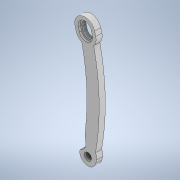
# Autodesk Inventor part: Part2
Saved by Autodesk Inventor 2020.3 (Build 243373000, 373)
## iProperties
Created: 2019-08-12
Part Number: Part2
Material: Generic
Document SubType Name: Modeling
Designer: Horváth Patrik
Density: 1 g/cm^3
Appearance: Default
Author: Horváth Patrik
Autodesk Inventor part; units mm, degrees
ref_plane "YZ Plane" through (0, 0, 0) normal (1, 0, 0) x (0, 1, 0)
ref_plane "XZ Plane" through (0, 0, 0) normal (0, 1, 0) x (-1, 0, 0)
ref_plane "XY Plane" through (0, 0, 0) normal (0, 0, 1) x (1, 0, 0)
ref_plane "Work Plane1" through (-0.0405, 69.8618, 0) normal (0, 0, 1) x (0.6413599, 0.7672402, 0)
ref_plane "Work Plane3" through (5.5931, 11.378, 1) normal (0, 0, 1) x (1, 0, 0)
sketch "Sketch2" plane through (5.5931, 11.378, 1) normal (0, 0, 1) x (1, 0, 0)
  arc A0 (-2.9323, 0.6339) -> (-4.1247, 52.0744) centre (-110.4489, 23.8756) ccw projected
  arc A1 (2.9323, -0.6339) -> (1.6748, 53.6125) centre (-110.4489, 23.8756) ccw projected
  arc A2 (1.6748, 53.6125) -> (-4.1247, 52.0744) centre (-1.225, 52.8435) ccw projected
  circle A3 centre (0, 0) radius 3 projected
  circle A4 centre (0, 0) radius 1.25 projected
  circle A5 centre (-1.225, 52.8435) radius 3 projected
  circle A6 centre (-1.225, 52.8435) radius 1.4795 projected
  point P0 (-5.5931, -11.378)
  point P1 (-2.9323, 0.6339)
  point P2 (2.9323, -0.6339)
extrude "Extrusion2" add sketch "Sketch2" along normal blind 3
ref_plane "Work Plane6" through (4.3681, 64.2214, 5) normal (0, 0, 1) x (1, 0, 0)
sketch "Sketch4" plane through (4.3681, 64.2214, 4) normal (0, 0, 1) x (1, 0, 0)
  arc A0 (4.1572, -53.4773) -> (2.8997, 0.7691) centre (-109.2239, -28.9678) ccw construction
  arc A1 (-1.7073, -52.2096) -> (-2.8997, -0.7691) centre (-109.2239, -28.9678) ccw construction
  circle A2 centre (0, 0) radius 3 construction
  circle A3 centre (0, 0) radius 3 construction
  circle A4 centre (0, 0) radius 1.4795 construction
  arc A5 (0.2521, -0.9677) -> (-0.2606, 0.9654) centre (-109.2239, -28.9678) ccw construction
  arc A6 (5.0961, 0.2712) -> (4.5608, 2.2899) centre (-109.2239, -28.9678) ccw
  arc A7 (-4.592, -2.2067) -> (-5.082, -0.359) centre (-109.2239, -28.9678) ccw
  arc A8 (-4.592, -2.2067) -> (5.0961, 0.2712) centre (0.2521, -0.9677) ccw
  arc A9 (4.5608, 2.2899) -> (-5.082, -0.359) centre (-0.2606, 0.9654) ccw
  arc A10 (-1.7073, -52.2096) -> (4.1572, -53.4773) centre (1.225, -52.8435) ccw projected
  arc A11 (2.8997, 0.7691) -> (-2.8997, -0.7691) centre (0, 0) ccw projected
  arc A12 (-1.7073, -52.2096) -> (-2.8997, -0.7691) centre (-109.2239, -28.9678) ccw projected
  point P0 (-4.3681, -64.2214)
  dimension "d16" = 10
  dimension "d26" = 1
  dimension "d27" = 1
  constraints: 11 point on circle, 5 centre point, 4 tangent, 2 coincident, 2 concentric
  measures "d16" radial gap between concentric circles of A7 A6
  measures "d26" distance of point (0, 0) A5.end
  measures "d27" distance of A5.start point (0, 0)
extrude "Extrusion4" add sketch "Sketch4" against normal blind 3
ref_plane "Work Plane7" through (5.5931, 11.378, 5) normal (0, 0, 1) x (1, 0, 0)
sketch "Sketch5" plane through (5.5931, 11.378, 5) normal (0, 0, 1) x (1, 0, 0)
  arc A0 (-0.9646, 51.8435) -> (-1.4951, 53.8435) centre (-110.4489, 23.8756) ccw construction
  arc A1 (0.7309, 52.2766) -> (0.1923, 54.3076) centre (-110.4489, 23.8756) ccw
  arc A2 (-2.6602, 51.4103) -> (-3.1824, 53.3794) centre (-110.4489, 23.8756) ccw
  arc A3 (-2.6602, 51.4103) -> (0.7309, 52.2766) centre (-0.9646, 51.8435) ccw
  arc A4 (0.1923, 54.3076) -> (-3.1824, 53.3794) centre (-1.4951, 53.8435) ccw
  arc A5 (2.6687, 52.7716) -> (2.1206, 54.838) centre (-110.4489, 23.8756) ccw projected
  arc A6 (2.1206, 54.838) -> (-5.1108, 52.849) centre (-1.4951, 53.8435) ccw projected
  arc A7 (-4.598, 50.9153) -> (-5.1108, 52.849) centre (-110.4489, 23.8756) ccw projected
  arc A8 (-4.598, 50.9153) -> (2.6687, 52.7716) centre (-0.9646, 51.8435) ccw projected
  arc A9 (3.3358, 55.1334) -> (-6.307, 52.4844) centre (-1.4856, 53.8089) ccw projected
  arc A10 (3.8712, 53.1147) -> (3.3358, 55.1334) centre (-110.4489, 23.8756) ccw projected
  arc A11 (2.869, 48.6758) -> (3.8712, 53.1147) centre (-0.9729, 51.8758) ccw projected
  arc A12 (-5.817, 50.6368) -> (-2.9702, 47.292) centre (-0.9729, 51.8758) ccw projected
  arc A13 (-5.817, 50.6368) -> (-6.307, 52.4844) centre (-110.4489, 23.8756) ccw projected
  point P0 (-5.5931, -11.378)
  dimension "d12" = 3.5
  constraints: 10 point on circle, 5 centre point, 4 tangent, 2 coincident, 2 concentric
  measures "d12" radial gap between concentric circles of A1 A2
extrude "Extrusion5" cut sketch "Sketch5" against normal blind 5 contours A3 A2 A4 A1
sketch "Sketch7" plane through (5.5931, 11.378, 4) normal (0, 0, 1) x (1, 0, 0)
  circle A0 centre (0, 0) radius 1.25 projected
  circle A1 centre (0, 0) radius 1.8
  arc A2 (-3.9097, 0.8452) -> (3.9097, -0.8452) centre (0, 0) ccw
  arc A3 (4.2266, 0.621) -> (-3.5928, 2.3113) centre (0.3169, 1.4661) ccw
  arc A4 (-2.9323, 0.6339) -> (-2.9702, 47.292) centre (-110.4489, 23.8756) ccw projected
  arc A5 (2.9323, -0.6339) -> (2.869, 48.6758) centre (-110.4489, 23.8756) ccw projected
  line L0 (0.3169, 1.4661) -> (0, 0) construction
  line L1 (-3.5928, 2.3113) -> (-3.9097, 0.8452)
  line L2 (4.2266, 0.621) -> (3.9097, -0.8452)
  line L3 (-2.9323, 0.6339) -> (2.9323, -0.6339) construction
  point P0 (-5.5931, -11.378)
  dimension "d19" = 3.6
  dimension "d20" = 8
  dimension "d21" = 1.5
  constraints: 8 end point, 4 point on circle, 4 tangent, 3 centre point, 2 coincident, 1 equal radius, 1 perpendicular
  measures "d19" diameter of A1
  measures "d20" diameter of A2
  measures "d21" distance of L0.start L0.end
extrude "Extrusion6" cut sketch "Sketch7" against normal up to surface (3 mm away) contours A1
extrude "Extrusion7" add sketch "Sketch7" against normal up to surface (3 mm away) contours L1 A3 L2 A2
sketch "Sketch8" plane through (5.5931, 11.378, 4) normal (0, 0, 1) x (1, 0, 0)
  arc A0 (-2.6602, 51.4103) -> (-3.1824, 53.3794) centre (-110.4489, 23.8756) ccw projected
  arc A1 (0.1923, 54.3076) -> (-3.1824, 53.3794) centre (-1.4951, 53.8435) ccw projected
  arc A2 (0.7309, 52.2766) -> (0.1923, 54.3076) centre (-110.4489, 23.8756) ccw projected
  arc A3 (-2.6602, 51.4103) -> (0.7309, 52.2766) centre (-0.9646, 51.8435) ccw projected
  arc A4 (-3.3868, 51.2247) -> (-3.9056, 53.1805) centre (-110.4489, 23.8756) ccw
  arc A5 (-3.3868, 51.2247) -> (1.4576, 52.4622) centre (-0.9646, 51.8435) ccw
  arc A6 (1.4576, 52.4622) -> (0.9154, 54.5065) centre (-110.4489, 23.8756) ccw
  arc A7 (0.9154, 54.5065) -> (-3.9056, 53.1805) centre (-1.4951, 53.8435) ccw
  arc A8 (-4.162, 51.0267) -> (-4.6769, 52.9683) centre (-110.4489, 23.8756) ccw
  arc A9 (-4.162, 51.0267) -> (2.2327, 52.6602) centre (-0.9646, 51.8435) ccw
  arc A10 (2.2327, 52.6602) -> (1.6867, 54.7186) centre (-110.4489, 23.8756) ccw
  arc A11 (1.6867, 54.7186) -> (-4.6769, 52.9683) centre (-1.4951, 53.8435) ccw
  point P0 (-5.5931, -11.378)
  dimension "d31" = 2.5
  dimension "d32" = 0.8
  constraints: 16 point on circle, 8 centre point, 6 other
  measures "d31" radius of A7
  measures "d32" radial gap between concentric circles of A7 A11
extrude "Extrusion8" cut sketch "Sketch8" against normal up to surface (3 mm away) contours A4 A7 A6 A5
extrude "Extrusion9" cut sketch "Sketch8" against normal blind 1 contours A8 A11 A10 A9
sketch "Sketch9" plane through (5.5931, 11.378, 4) normal (0, 0, 1) x (1, 0, 0)
  arc A0 (-3.9097, 0.8452) -> (3.9097, -0.8452) centre (0, 0) ccw projected
  arc A1 (3.7507, 3.5177) -> (2.869, 48.6758) centre (-110.4489, 23.8756) ccw projected
  arc A2 (-4.162, 51.0267) -> (-4.6769, 52.9683) centre (-110.4489, 23.8756) ccw projected
  arc A3 (1.6867, 54.7186) -> (-4.6769, 52.9683) centre (-1.4951, 53.8435) ccw projected
  arc A4 (2.2327, 52.6602) -> (1.6867, 54.7186) centre (-110.4489, 23.8756) ccw projected
  arc A5 (-4.162, 51.0267) -> (2.2327, 52.6602) centre (-0.9646, 51.8435) ccw projected
  circle A6 centre (0, 0) radius 1.8 projected
  arc A7 (3.7507, 3.5177) -> (2.869, 48.6758) centre (-110.4489, 23.8756) ccw projected
  arc A8 (2.869, 48.6758) -> (3.8712, 53.1147) centre (-0.9729, 51.8758) ccw projected
  arc A9 (3.8712, 53.1147) -> (3.3358, 55.1334) centre (-110.4489, 23.8756) ccw projected
  arc A10 (3.3358, 55.1334) -> (-6.307, 52.4844) centre (-1.4856, 53.8089) ccw projected
  arc A11 (-5.817, 50.6368) -> (-6.307, 52.4844) centre (-110.4489, 23.8756) ccw projected
  arc A12 (-5.817, 50.6368) -> (-2.9702, 47.292) centre (-0.9729, 51.8758) ccw projected
  arc A13 (-2.148, 4.6164) -> (-2.9702, 47.292) centre (-110.4489, 23.8756) ccw projected
  arc A14 (-2.148, 4.6164) -> (-3.5928, 2.3113) centre (0.3169, 1.4661) ccw projected
  line L0 (-3.5928, 2.3113) -> (-3.9097, 0.8452) projected
  arc A15 (-3.9097, 0.8452) -> (3.9097, -0.8452) centre (0, 0) ccw projected
  line L1 (3.9097, -0.8452) -> (4.2266, 0.621) projected
  arc A16 (4.2266, 0.621) -> (3.7507, 3.5177) centre (0.3169, 1.4661) ccw projected
  arc A17 (-3.4806, 1.3307) -> (-3.9097, 0.8452) centre (-3.262, 0.7051) ccw
  arc A18 (-3.4806, 1.3307) -> (-1.0527, 5.3618) centre (-4.6968, 4.8099) ccw
  arc A19 (-2.148, 4.6164) -> (-2.9702, 47.292) centre (-110.4489, 23.8756) ccw projected
  arc A20 (-1.162, 11.3705) -> (-1.0527, 5.3618) centre (21.4998, 8.7774) ccw
  point P0 (-5.5931, -11.378)
  point P1 (3.7507, 3.5177)
  point P2 (-1.162, 11.3705)
  constraints: 7 point on circle, 4 tangent, 3 centre point
extrude "Extrusion10" cut sketch "Sketch9" against normal up to surface (3 mm away) contours L0 A14 A13 A20 A18 A17
body "Solid1"
